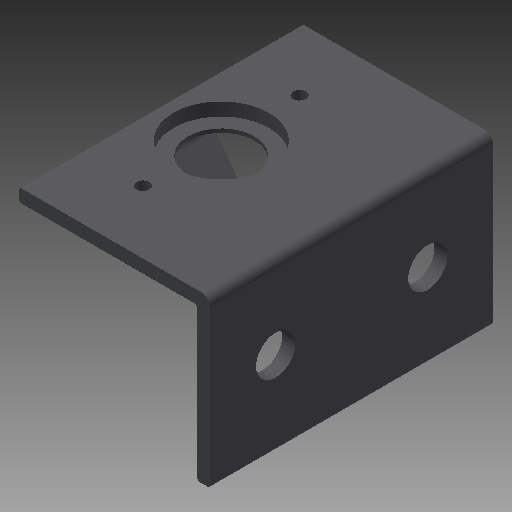
# Autodesk Inventor part: May Tec 1.64.5101._Mounting angle
Saved by Autodesk Inventor 2018 (Build 220112000, 112)
## iProperties
Category: PARTsolutions
Company: MAYTEC
Created: 2018-01-04
Part Number: May Tec 1.64.5101._Mounting angle
Catalog Web Link: www.cadenas.de
Description: 1.64.5101-Mounting angle
Vendor: MAYTEC
Document SubType Name: Modeling
Designer: psAdmin
Manufacturer: MAYTEC
Mass: 1.93898 g
Surface Area: 33.5104 cm^2
Volume: 1.93898 cm^3
Density: 1 g/cm^3
Material: Generic
Appearance: PSOLRGB-175-175-175
PSOL_IDENT_0: {$CADENAS_DATA\23d-libs\maytec\maytec_3d\anbauzubehoer\schnellverschluesse\montagewinkel\1.64.5101.p
PSOL_IDENT_1: rj},211 {VTYP=3D},{NB=May Tec 1.64.5101._Mounting angle},{LINA=May Tec 1.64.5101._Mounting angle},{N
PSOL_IDENT_2: N=1.64.5101},{DATE=09.02.2017 10:28:50},{GEOMDATE=17.01.2013 11:15:00},{VERSION=},{LINEID=10},{LINES
PSOL_IDENT_3: UBID=-1},{WBVAR=}  {NB=May Tec 1.64.5101._Mounting angle},{LINA=May Tec 1.64.5101._Mounting angle},{
PSOL_IDENT_4: KT=DUMMY},{PARTNR=1.64.5101},{DESCRIPTION=Montagewinkel},{XTRANS=Mounting angle}
NN: 1.64.5101
NT: Mounting angle
NB: May Tec 1.64.5101._Mounting angle
NBSYN: May Tec $PARTNR.._$XTRANS.
LINA: May Tec 1.64.5101._Mounting angle
PARTNR: 1.64.5101
DESCRIPTION: Mounting angle
SUPPLIER: MAYTEC
ARTICLENO: May Tec 1.64.5101._Mounting angle
BOMINFO: May Tec 1.64.5101._Mounting angle
CREATOR: CADENAS GmbH
Title: May Tec 1.64.5101._Mounting angle
Author: Cadenas PARTsolutions
Comments: Mounting angle
Autodesk Inventor part; units mm, degrees
sketch "Skizze_1" plane through (0, 0, 0) normal (0, 0, 1) x (1, 0, 0)
  line L0 (0, -0.3) -> (0, -1.2)
  arc A0 (0, -1.2) -> (0.3, -1.5) centre (0.3, -1.2) ccw
  line L1 (0.3, -1.5) -> (20.2, -1.5)
  arc A1 (20.5, -1.8) -> (20.2, -1.5) centre (20.2, -1.8) ccw
  line L2 (20.5, -1.8) -> (20.5, -18.7)
  arc A2 (20.5, -18.7) -> (20.8, -19) centre (20.8, -18.7) ccw
  line L3 (20.8, -19) -> (21.7, -19)
  arc A3 (21.7, -19) -> (22, -18.7) centre (21.7, -18.7) ccw
  line L4 (22, -18.7) -> (22, -1)
  arc A4 (22, -1) -> (21, 0) centre (21, -1) ccw
  line L5 (21, 0) -> (0.3, 0)
  arc A5 (0.3, 0) -> (0, -0.3) centre (0.3, -0.3) ccw
  constraints: 12 end point, 12 point on circle, 6 centre point
extrude "Extrusion1" add sketch "Skizze_1" along normal mid plane 32.5
sketch "Skizze_2" plane through (22, 0, 0) normal (1, 0, 0) x (0, 0, -1)
  circle A0 centre (8.75, -9.5) radius 2.25
  constraints: 1 centre point
extrude "Extrusion2" cut sketch "Skizze_2" along normal mid plane 3
sketch "Skizze_3" plane through (22, 0, 0) normal (1, 0, 0) x (0, 0, -1)
  circle A0 centre (-8.75, -9.5) radius 2.25
  constraints: 1 centre point
extrude "Extrusion3" cut sketch "Skizze_3" along normal mid plane 3
sketch "Skizze_4" plane through (0, 0, 0) normal (0, 0, 1) x (1, 0, 0)
  arc A0 (2.1852, -1.45) -> (0.5463, -5.08) centre (2.1852, -3.635) ccw
  line L0 (0.5463, -5.08) -> (5.946, -10.1545)
  arc A1 (5.4062, -11.35) -> (5.946, -10.1545) centre (5.4062, -10.6304) ccw
  line L1 (5.4062, -11.35) -> (4, -11.35)
  line L2 (4, -11.35) -> (4, -11.8)
  line L3 (4, -11.8) -> (5.3389, -11.8)
  arc A2 (5.3389, -11.8) -> (6.239, -9.8064) centre (5.3389, -10.6) ccw
  line L4 (6.239, -9.8064) -> (0.8838, -4.7824)
  arc A3 (2.1852, -1.9) -> (0.8838, -4.7824) centre (2.1852, -3.635) ccw
  line L5 (2.1852, -1.9) -> (11.8148, -1.9)
  arc A4 (13.1162, -4.7824) -> (11.8148, -1.9) centre (11.8148, -3.635) ccw
  line L6 (13.1162, -4.7824) -> (7.761, -9.8064)
  arc A5 (7.761, -9.8064) -> (8.6611, -11.8) centre (8.6611, -10.6) ccw
  line L7 (8.6611, -11.8) -> (10, -11.8)
  line L8 (10, -11.8) -> (10, -11.35)
  line L9 (10, -11.35) -> (8.5938, -11.35)
  arc A6 (8.054, -10.1545) -> (8.5938, -11.35) centre (8.5938, -10.6304) ccw
  line L10 (8.054, -10.1545) -> (13.4537, -5.08)
  arc A7 (13.4537, -5.08) -> (11.8148, -1.45) centre (11.8148, -3.635) ccw
  line L11 (11.8148, -1.45) -> (2.1852, -1.45)
  constraints: 24 end point, 16 point on circle, 8 centre point
extrude "Extrusion4" add sketch "Skizze_4" along normal mid plane 12
sketch "Skizze_5" plane through (0, 0, 0) normal (0, 1, 0) x (-1, 0, 0)
  line L0 (-1.809, 5.7484) -> (-2.5923, 9.8744)
  arc A0 (-2.5923, 9.8744) -> (-6.2765, 12.925) centre (-6.2765, 9.175) ccw
  line L1 (-6.2765, 12.925) -> (-7.7235, 12.925)
  arc A1 (-7.7235, 12.925) -> (-11.4077, 9.8744) centre (-7.7235, 9.175) ccw
  line L2 (-11.4077, 9.8744) -> (-12.191, 5.7484)
  line L3 (-12.191, 5.7484) -> (-12.191, -5.7484)
  line L4 (-12.191, -5.7484) -> (-11.4077, -9.8744)
  arc A2 (-11.4077, -9.8744) -> (-7.7235, -12.925) centre (-7.7235, -9.175) ccw
  line L5 (-7.7235, -12.925) -> (-6.2765, -12.925)
  arc A3 (-6.2765, -12.925) -> (-2.5923, -9.8744) centre (-6.2765, -9.175) ccw
  line L6 (-2.5923, -9.8744) -> (-1.809, -5.7484)
  line L7 (-1.809, -5.7484) -> (-1.809, 5.7484)
  constraints: 16 end point, 8 point on circle, 4 centre point
extrude "Extrusion5" add sketch "Skizze_5" against normal blind 1.94
sketch "Skizze_6_ALT_Drilling_1" plane through (0, 0, 0) normal (0, 1, 0) x (-1, 0, 0)
  circle A0 centre (-7, 0) radius 5.5
  constraints: 1 centre point
extrude "Extrusion6" cut sketch "Skizze_6_ALT_Drilling_1" against normal blind 1.5
sketch "Skizze_7_ALT_Drilling_2" plane through (0, 0, 0) normal (0, 1, 0) x (-1, 0, 0)
  circle A0 centre (-7, 0) radius 3.825
  constraints: 1 centre point
extrude "Extrusion7" cut sketch "Skizze_7_ALT_Drilling_2" against normal blind 2.6
sketch "Skizze_8" plane through (17, 0, 0) normal (1, 0, 0) x (0, 0, -1)
  line L0 (-6, -1.94) -> (-6, -12.9)
  line L1 (-6, -12.9) -> (-3.9, -12.9)
  line L2 (-3.9, -12.9) -> (-6, -1.94)
  constraints: 6 end point
extrude "Extrusion8" cut sketch "Skizze_8" against normal blind 30
sketch "Skizze_9" plane through (17, 0, 0) normal (1, 0, 0) x (0, 0, -1)
  line L0 (3.9, -12.9) -> (6, -12.9)
  line L1 (6, -12.9) -> (6, -1.94)
  line L2 (6, -1.94) -> (3.9, -12.9)
  constraints: 6 end point
extrude "Extrusion9" cut sketch "Skizze_9" against normal blind 30
sketch "Skizze_10_ALT_Drilling_3" plane through (0, 0, 0) normal (0, 1, 0) x (-1, 0, 0)
  circle A0 centre (-7, 9) radius 0.75
  constraints: 1 centre point
extrude "Extrusion10" cut sketch "Skizze_10_ALT_Drilling_3" against normal blind 3
sketch "Skizze_11_ALT_Drilling_4" plane through (0, 0, 0) normal (0, 1, 0) x (-1, 0, 0)
  circle A0 centre (-7, -9) radius 0.75
  constraints: 1 centre point
extrude "Extrusion11" cut sketch "Skizze_11_ALT_Drilling_4" against normal blind 3
sketch "Skizze_12" plane through (0, -11.8, 0) normal (0, 1, 0) x (1, 0, 0)
  line L0 (3, -5.05) -> (11, -5.05)
  line L1 (11, -5.05) -> (11, 5.05)
  line L2 (11, 5.05) -> (3, 5.05)
  line L3 (3, 5.05) -> (3, -5.05)
  arc A0 (4, -2.55) -> (5.5, -4.05) centre (5.5, -2.55) ccw
  line L4 (5.5, -4.05) -> (8.5, -4.05)
  arc A1 (8.5, -4.05) -> (10, -2.55) centre (8.5, -2.55) ccw
  line L5 (10, -2.55) -> (10, 2.55)
  arc A2 (10, 2.55) -> (8.5, 4.05) centre (8.5, 2.55) ccw
  line L6 (8.5, 4.05) -> (5.5, 4.05)
  arc A3 (5.5, 4.05) -> (4, 2.55) centre (5.5, 2.55) ccw
  line L7 (4, 2.55) -> (4, -2.55)
  constraints: 16 end point, 8 point on circle, 4 centre point
extrude "Extrusion12" cut sketch "Skizze_12" along normal blind 0.45
ref_plane "side_1_XY" through (22, -9.5, 0) normal (1, 0, 0) x (0, 1, 0)
ref_plane "side_1_YZ" through (22, -9.5, 0) normal (0, 1, 0) x (0, 0, 1)
ref_plane "side_1_ZX" through (22, -9.5, 0) normal (0, 0, 1) x (1, 0, 0)
ref_plane "side_2_XY" through (7, -1.6, 0) normal (0, 1, 0) x (1, 0, 0)
ref_plane "side_2_YZ" through (7, -1.6, 0) normal (1, 0, 0) x (0, 0, -1)
ref_plane "side_2_ZX" through (7, -1.6, 0) normal (0, 0, -1) x (0, 1, 0)
body "Solid1"
